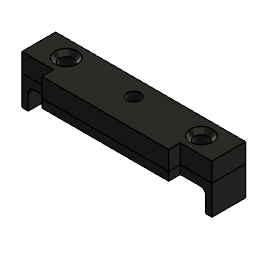
Kicker Bar v1 (Autodesk Fusion 360 design; units mm, degrees)
Autodesk Fusion 360 part; units mm, degrees
sketch "Sketch1" plane through (0, 0, 0) normal (0, 1, 0) x (1, 0, 0)
  circle A0 centre (0, 0) radius 1.55
  line L0 (22.5, 4) -> (-22.5, 4)
  line L1 (-22.5, 4) -> (-22.5, -4)
  line L2 (-22.5, -4) -> (22.5, -4)
  line L3 (22.5, -4) -> (22.5, 4)
  line L4 (22.5, 4) -> (-22.5, -4) construction
  line L5 (-22.5, 4) -> (22.5, -4) construction
  line L6 (0, 0) -> (-16, 0)
  circle A1 centre (-16, 0) radius 1.65
  line L7 (0, -4) -> (0, 4) construction
  circle A2 centre (16, 0) radius 1.65
  dimension "d1" = 3.1
  dimension "d2" = 45
  dimension "d3" = 8
  dimension "d4" = 3.3
  dimension "d20" = 16
  constraint coincident A0.centre L6.start
  constraint horizontal L0
  constraint perpendicular L0 L1
  constraint parallel L0 L2
  constraint parallel L1 L3
  constraint coincident L4 A0.centre
  constraint coincident L5 A0.centre
  constraint horizontal L6
  constraint coincident L6.end A1.centre
  constraint midpoint L2 L7.start
  constraint midpoint L0 L7.end
  constraint symmetric A1 L7 A2
  measures "d1" diameter of A0
  measures "d2" distance of L1.end L2.end
  measures "d3" distance of L0.end L1.end
  measures "d4" diameter of A1
  measures "d20" distance of A0.centre L6.end
extrude "Extrude1" add sketch "Sketch1" along normal blind 4.5 makes body 1
chamfer "Chamfer1" distance 1 angle 45 2 edges at (-17.5383, 4.5, -0.5967) (14.4617, 4.5, -0.5967) on bodies 1
ref_plane "WorkPlane1" through (0, -1, 0) normal (0, -1, 0) x (-1, 0, 0)
sketch "Sketch2" plane through (0, -1, 0) normal (0, -1, 0) x (-1, 0, 0)
  circle A0 centre (0, 0) radius 1.6
  line L0 (0, 0) -> (-16, 0)
  circle A1 centre (16, 0) radius 1.65
  circle A2 centre (-16, 0) radius 1.65
  line L1 (22.5, -4) -> (-22.5, -4)
  line L2 (-22.5, -4) -> (-22.5, 4)
  line L3 (-22.5, 4) -> (22.5, 4)
  line L4 (22.5, 4) -> (22.5, -4)
  line L5 (22.5, -4) -> (-22.5, 4) construction
  line L6 (-22.5, -4) -> (22.5, 4) construction
  line L7 (0, 0) -> (16, 0)
  line L8 (0, 0) -> (-16, 0)
  dimension "d9" = 3.2
  dimension "d10" = 3.3
  dimension "d11" = 3.3
  dimension "d22" = 16
  dimension "d23" = 16
  dimension "d24" = 45
  dimension "d25" = 8
  constraint coincident A0.centre L0.start
  constraint horizontal L0
  constraint coincident L0.end A2.centre
  constraint horizontal L1
  constraint perpendicular L1 L2
  constraint parallel L1 L3
  constraint parallel L2 L4
  constraint coincident L5 A0.centre
  constraint coincident L6 A0.centre
  constraint coincident A1.centre L7.end
  measures "d9" diameter of A0
  measures "d10" diameter of A1
  measures "d11" diameter of A2
  measures "d22" distance of A0.centre A1.centre
  measures "d23" distance of A0.centre L0.end
  measures "d24" distance of L1.start L1.end
  measures "d25" distance of L1.start L3.end
extrude "Extrude2" add sketch "Sketch2" along normal blind 3 separate body makes body 2
sketch "Sketch3" plane through (0, -4, 0) normal (0, -1, 0) x (1, 0, 0)
  circle A0 centre (0, 0) radius 1.6
  circle A1 centre (16, 0) radius 1.65
  circle A2 centre (-16, 0) radius 1.65
  line L0 (-22.5, -4) -> (22.5, -4)
  line L1 (22.5, -4) -> (22.5, 4)
  line L2 (22.5, 4) -> (-22.5, 4)
  line L3 (-22.5, 4) -> (-22.5, -4)
  line L4 (-19.2, 0) -> (-17.6, -2.7713)
  line L5 (-17.6, -2.7713) -> (-14.4, -2.7713)
  line L6 (-14.4, -2.7713) -> (-12.8, 0)
  line L7 (-12.8, 0) -> (-14.4, 2.7713)
  line L8 (-14.4, 2.7713) -> (-17.6, 2.7713)
  line L9 (-17.6, 2.7713) -> (-19.2, 0)
  line L10 (0, -4) -> (0, 4) construction
  line L11 (14.4, -2.7713) -> (12.8, 0)
  line L12 (12.8, 0) -> (14.4, 2.7713)
  line L13 (14.4, 2.7713) -> (17.6, 2.7713)
  line L14 (17.6, 2.7713) -> (19.2, 0)
  line L15 (19.2, 0) -> (17.6, -2.7713)
  line L16 (17.6, -2.7713) -> (14.4, -2.7713)
  point P0 (-16, 0)
  dimension "d14" = 3.2
  constraint coincident P0 A2.centre
  constraint midpoint L0 L10.start
  constraint midpoint L2 L10.end
  constraint symmetric L4.start L10 L14.end
  constraint symmetric L4.end L10 L15.end
  constraint symmetric L5.end L10 L11.start
  constraint symmetric L6.end L10 L11.end
  constraint symmetric L7.end L10 L12.end
  constraint symmetric L8.end L10 L13.end
  measures "d14" distance of L4.start P0
extrude "Extrude3" cut sketch "Sketch3" against normal blind 2 contours L4 L5 L6 L7 L8 L9 | L11 L12 L13 L14 L15 L16 bodies 2
sketch "Sketch4" plane through (0, -1, 0) normal (0, 1, 0) x (-1, 0, 0)
  circle A0 centre (0, 0) radius 1.6
  circle A1 centre (-16, 0) radius 1.65
  circle A2 centre (16, 0) radius 1.65
  line L0 (-22.5, -4) -> (22.5, -4)
  line L1 (22.5, -4) -> (22.5, 4)
  line L2 (22.5, 4) -> (-22.5, 4)
  line L3 (-22.5, 4) -> (-22.5, -4)
  circle A3 centre (0, 0) radius 3.6
  dimension "d17" = 7.2
  constraint coincident A0.centre A3.centre
  measures "d17" diameter of A3
extrude "Extrude4" add sketch "Sketch4" along normal blind 1 contours L0 L1 L2 L3 bodies 2
sketch "Sketch5" plane through (0, 0, 0) normal (0, -1, 0) x (1, 0, 0)
  circle A0 centre (0, 0) radius 1.55
  circle A1 centre (16, 0) radius 1.65
  circle A2 centre (-16, 0) radius 1.65
  line L0 (22.5, -4) -> (22.5, 4)
  line L1 (22.5, 4) -> (-22.5, 4)
  line L2 (-22.5, 4) -> (-22.5, -4)
  line L3 (-22.5, -4) -> (22.5, -4)
  line L4 (0, 4) -> (0, 6.75)
  line L5 (15, 6.75) -> (-15, 6.75)
  line L6 (15, 6.75) -> (15, 4)
  line L7 (-15, 6.75) -> (-15, 4)
  dimension "d26" = 2.75
  dimension "d27" = 30
  constraint midpoint L1 L4.start
  constraint perpendicular L1 L4
  constraint midpoint L4.end L5
  constraint perpendicular L4 L5
  constraint coincident L1 L6.end
  constraint perpendicular L1 L6
  constraint coincident L1 L7.end
  constraint perpendicular L1 L7
  measures "d26" distance of L4.start L4.end
  measures "d27" distance of L5.start L5.end
extrude "Extrude5" add sketch "Sketch5" against normal blind 4.5 contours L1 L4 L5 L6 | L1 L4 L5 L7 bodies 1
sketch "Sketch6" plane through (0, -4, 0) normal (0, -1, 0) x (1, 0, 0)
  line L0 (17.6, 2.7713) -> (19.2, 0)
  line L1 (19.2, 0) -> (17.6, -2.7713)
  line L2 (17.6, -2.7713) -> (14.4, -2.7713)
  line L3 (14.4, -2.7713) -> (12.8, 0)
  line L4 (12.8, 0) -> (14.4, 2.7713)
  line L5 (14.4, 2.7713) -> (17.6, 2.7713)
  line L6 (-17.6, -2.7713) -> (-19.2, 0)
  line L7 (-19.2, 0) -> (-17.6, 2.7713)
  line L8 (-17.6, 2.7713) -> (-14.4, 2.7713)
  line L9 (-14.4, 2.7713) -> (-12.8, 0)
  line L10 (-12.8, 0) -> (-14.4, -2.7713)
  line L11 (-14.4, -2.7713) -> (-17.6, -2.7713)
  circle A0 centre (0, 0) radius 1.6
  line L12 (-22.5, -4) -> (22.5, -4)
  line L13 (22.5, -4) -> (22.5, 4)
  line L14 (22.5, 4) -> (-22.5, 4)
  line L15 (-22.5, 4) -> (-22.5, -4)
  line L16 (0, 4) -> (0, 6.75)
  line L17 (-15, 6.75) -> (15, 6.75)
  line L18 (15, 6.75) -> (15, 4)
  line L19 (-15, 6.75) -> (-15, 4)
  dimension "d30" = 2.75
  dimension "d31" = 30
  constraint midpoint L14 L16.start
  constraint perpendicular L14 L16
  constraint midpoint L16.end L17
  constraint perpendicular L16 L17
  constraint coincident L14 L18.end
  constraint perpendicular L14 L18
  constraint coincident L14 L19.end
  constraint perpendicular L14 L19
  measures "d30" distance of L16.start L16.end
  measures "d31" distance of L17.start L17.end
extrude "Extrude6" add sketch "Sketch6" against normal blind 4 contours L14 L16 L17 L19 | L14 L16 L17 L18 bodies 2
extrude "Extrude7" cut 1 faces at (0.0399, -4, 5.0318) along direction (0, 1, 0) blind 2 on bodies 2 bodies 2
extrude "Extrude8" cut sketch "Sketch3" against normal blind 3 contours L4 L5 L6 L7 L8 L9 | L11 L12 L13 L14 L15 L16 bodies 2
sketch "Sketch7" plane through (0, -2, 0) normal (0, -1, 0) x (1, 0, 0)
  line L0 (17.6, 2.7713) -> (19.2, 0)
  line L1 (19.2, 0) -> (17.6, -2.7713)
  line L2 (17.6, -2.7713) -> (14.4, -2.7713)
  line L3 (14.4, -2.7713) -> (12.8, 0)
  line L4 (12.8, 0) -> (14.4, 2.7713)
  line L5 (14.4, 2.7713) -> (17.6, 2.7713)
  line L6 (-17.6, -2.7713) -> (-19.2, 0)
  line L7 (-19.2, 0) -> (-17.6, 2.7713)
  line L8 (-17.6, 2.7713) -> (-14.4, 2.7713)
  line L9 (-14.4, 2.7713) -> (-12.8, 0)
  line L10 (-12.8, 0) -> (-14.4, -2.7713)
  line L11 (-14.4, -2.7713) -> (-17.6, -2.7713)
  circle A0 centre (0, 0) radius 1.6
  line L12 (-22.5, -4) -> (22.5, -4)
  line L13 (22.5, -4) -> (22.5, 4)
  line L14 (22.5, 4) -> (15, 4)
  line L15 (15, 4) -> (15, 6.75)
  line L16 (15, 6.75) -> (-15, 6.75)
  line L17 (-15, 6.75) -> (-15, 4)
  line L18 (-15, 4) -> (-22.5, 4)
  line L19 (-22.5, 4) -> (-22.5, -4)
  line L20 (-22.5, 4) -> (-21, 4)
  line L21 (-21, 4) -> (-21, -4)
  line L22 (-21, -4) -> (-22.5, -4)
  line L23 (-22.5, -4) -> (-22.5, 4)
  line L24 (22.5, 4) -> (21, 4)
  line L25 (21, 4) -> (21, -4)
  line L26 (21, -4) -> (22.5, -4)
  line L27 (22.5, -4) -> (22.5, 4)
  dimension "d38" = 1.5
  dimension "d39" = 1.5
  constraint horizontal L20
  constraint vertical L21
  constraint horizontal L22
  constraint vertical L23
  constraint coincident L18.end L19.start
  constraint horizontal L24
  constraint vertical L25
  constraint horizontal L26
  constraint vertical L27
  constraint coincident L12 L25.end
  constraint coincident L13.end L14.start
  measures "d38" distance of L18.end L20.end
  measures "d39" distance of L13.end L24.end
extrude "Extrude9" add sketch "Sketch7" along normal blind 5 contours L12 L18 L19 L20 L21 L22 L23 | L12 L13 L14 L24 L25 L26 L27 bodies 2
fillet "Fillet1" radius 1.25 2 edges at (-21, -2, 0) (21, -2, 0) on bodies 2
